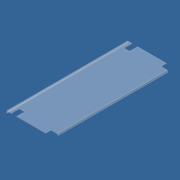
# Autodesk Inventor part: GE-12060
Saved by Autodesk Inventor 2012 (Build 160160000, 160)
## iProperties
Created: 2011-10-28
Part Number: GE-12060
Document SubType Name: Modeling
Designer: mcyr
Density: 1 g/cm^3
Description: Human Player Station Guard
Material: Default
Title: Human Player Station Guard
Author: mcyr
Autodesk Inventor part; units mm, degrees
ref_plane "YZ Plane" through (0, 0, 0) normal (1, 0, 0) x (0, 1, 0)
ref_plane "XZ Plane" through (0, 0, 0) normal (0, 1, 0) x (-1, 0, 0)
ref_plane "XY Plane" through (0, 0, 0) normal (0, 0, 1) x (1, 0, 0)
sketch "Sketch1" plane through (0, 0, 0) normal (0, 0, 1) x (1, 0, 0)
  line L0 (0, 0) -> (0, 20.955)
  line L1 (4.445, 25.4) -> (505.6861, 25.4)
  line L2 (0, 0) -> (6.35, 0)
  line L3 (6.35, 0) -> (6.35, 15.875)
  line L4 (9.525, 19.05) -> (503.0416, 19.05)
  arc A0 (9.525, 19.05) -> (6.35, 15.875) centre (9.525, 15.875) ccw
  arc A1 (4.445, 25.4) -> (0, 20.955) centre (4.445, 20.955) ccw
  line L5 (509.3272, 23.5045) -> (519.0883, 9.5642)
  line L6 (505.6424, 17.6961) -> (513.8867, 5.922)
  arc A2 (509.3272, 23.5045) -> (505.6861, 25.4) centre (505.6861, 20.955) ccw
  arc A3 (505.6424, 17.6961) -> (503.0416, 19.05) centre (503.0416, 15.875) ccw
  line L7 (513.8867, 5.922) -> (519.0883, 9.5642)
  point P0 (0, 25.4)
  point P1 (508, 25.4)
  point P2 (0, 22.225)
  point P3 (3.175, 25.4)
  dimension "d0" = 508
  dimension "d1" = 25.4
  dimension "d2" = 6.35
  dimension "d3" = 6.35
  dimension "d26" = 90
  dimension "d33" = 4.445
  dimension "d35" = 6.35
  dimension "d36" = 125
  dimension "d37" = 4.445
  dimension "d38" = 3.175
  dimension "d41" = 17.018
  constraints: 16 end point, 8 point on circle, 8 point on line, 8 tangent, 4 centre point, 2 parallel, 2 perpendicular, 1 vertical
  measures "d0" distance of point (0, 25.4) point (508, 25.4)
  measures "d1" distance of L0.start point (0, 25.4)
  measures "d2" distance between parallel lines of L0 L3
  measures "d3" distance between parallel lines of L1 L4
  measures "d26" angle of L4 L3
  measures "d33" radius of A1
  measures "d35" distance between parallel lines of L6 L5
  measures "d36" angle of L6 L4
  measures "d37" radius of A2
  measures "d38" radius of A3
  measures "d41" distance of L5.start L5.end
extrude "Extrusion4" add sketch "Sketch1" along normal blind 1352.55
sketch "Sketch4" plane through (4.445, 25.4, 0) normal (0, 1, 0) x (1, 0, 0)
  line L0 (0, -1352.55) -> (501.2411, -1352.55) projected
  line L1 (0, 0) -> (501.2411, 0) projected
  line L2 (-4.445, 0) -> (-4.445, -1352.55) projected
  line L3 (514.6433, 0) -> (514.6433, -1352.55) projected
  line L4 (46.355, 0) -> (109.855, 0)
  line L5 (109.855, 0) -> (109.855, -88.9)
  line L6 (109.855, -88.9) -> (46.355, -88.9)
  line L7 (46.355, -88.9) -> (46.355, 0)
  line L8 (46.355, -1352.55) -> (109.855, -1352.55)
  line L9 (109.855, -1352.55) -> (109.855, -1263.65)
  line L10 (109.855, -1263.65) -> (46.355, -1263.65)
  line L11 (46.355, -1263.65) -> (46.355, -1352.55)
  dimension "d44" = 63.5
  dimension "d45" = 88.9
  dimension "d46" = 50.8
  dimension "d47" = 88.9
  dimension "d48" = 50.8
  dimension "d49" = 63.5
  constraints: 16 end point, 4 parallel, 2 horizontal, 2 perpendicular, 2 point on line
  measures "d44" distance of L4.start L4.end
  measures "d45" distance between parallel lines of L6 L1
  measures "d46" distance of L4.start L2.start
  measures "d47" distance of L10.end L8.start
  measures "d48" distance of L8.start L2.end
  measures "d49" distance of L8.start L8.end
extrude "Extrusion5" cut sketch "Sketch4" against normal blind 12.7
sketch "Sketch5" plane through (505.6861, 25.4, 1352.55) normal (0, 1, 0) x (1, 0, 0)
  line L0 (-391.3861, 0) -> (0, 0) projected
  line L1 (-391.3861, 1352.55) -> (0, 1352.55) projected
  line L2 (13.4023, 1352.55) -> (13.4023, 0) projected
  line L3 (-69.5716, 0) -> (14.7564, 0)
  line L4 (14.7564, 0) -> (14.7564, 60.325)
  line L5 (14.7564, 60.325) -> (-69.5716, 60.325)
  line L6 (-69.5716, 60.325) -> (-69.5716, 0)
  line L7 (14.7422, 1352.55) -> (-69.5858, 1352.55)
  line L8 (-69.5858, 1352.55) -> (-69.5858, 1292.225)
  line L9 (-69.5858, 1292.225) -> (14.7422, 1292.225)
  line L10 (14.7422, 1292.225) -> (14.7422, 1352.55)
  point P0 (-505.6861, 1352.55)
  dimension "d52" = 84.328
  dimension "d53" = 60.325
  dimension "d55" = 60.325
  dimension "d56" = 84.328
  constraints: 16 end point, 4 parallel, 2 horizontal, 2 perpendicular, 2 point on line
  measures "d52" distance between parallel lines of L4 L6
  measures "d53" distance of L3.end L4.end
  measures "d55" distance of L9.end L7.start
  measures "d56" distance between parallel lines of L10 L8
extrude "Extrusion6" cut sketch "Sketch5" against normal blind 50.8
body "Solid2"
